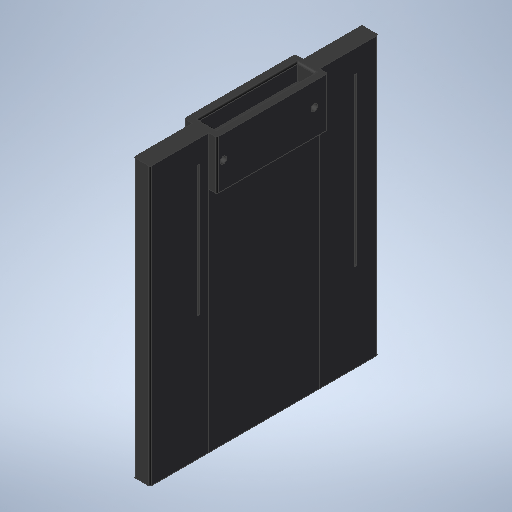
# Autodesk Inventor part: Chassis_Lower_Portion
Saved by Autodesk Inventor 2025 (Build 290162000, 162)
## iProperties
Created: 2024-06-26
Part Number: Chassis_Lower_Portion
Material: Generic
Document SubType Name: Modeling
Designer: sml6042
Density: 1 g/cm^3
Appearance: Default
Author: sml6042
Autodesk Inventor part; units mm, degrees
ref_plane "YZ Plane" through (0, 0, 0) normal (1, 0, 0) x (0, 1, 0)
ref_plane "XZ Plane" through (0, 0, 0) normal (0, 1, 0) x (-1, 0, 0)
ref_plane "XY Plane" through (0, 0, 0) normal (0, 0, 1) x (1, 0, 0)
sketch "Sketch1" plane through (0, 0, 0) normal (1, 0, 0) x (0, 1, 0)
  line L0 (0, 0) -> (0, -70)
  line L1 (0, -70) -> (-85, -70)
  line L2 (-85, -70) -> (-85, 0)
  line L3 (-85, 0) -> (0, 0)
  dimension "d0" = 70
  dimension "d1" = 85
  constraints: 8 end point, 3 perpendicular, 1 vertical
  measures "d0" distance of L0.start L0.end
  measures "d1" distance of L0.end L1.end
extrude "Extrusion1" add sketch "Sketch1" along normal blind 10
sketch "Sketch2" plane through (0, 0, 0) normal (0, 1, 0) x (1, 0, 0)
  line L0 (0, 0) -> (0, 70) projected
  line L1 (0, 0) -> (0, 20.125)
  line L2 (0, 20.125) -> (2.38, 20.125)
  line L3 (2.38, 20.125) -> (2.38, 50.375)
  line L4 (2.38, 50.375) -> (7.63, 50.375)
  line L5 (7.63, 50.375) -> (7.63, 20.125)
  line L6 (7.63, 20.125) -> (2.38, 20.125)
  dimension "d4" = 20.125
  dimension "d5" = 2.38
  dimension "d6" = 30.25
  dimension "d7" = 5.25
  constraints: 12 end point, 4 perpendicular, 2 point on line, 1 horizontal
  measures "d4" distance of L0.start L1.end
  measures "d5" distance of L1.end L2.end
  measures "d6" distance of L2.end L3.end
  measures "d7" distance of L3.end L4.end
extrude "Extrusion2" cut sketch "Sketch2" against normal blind 5.1
sketch "Sketch3" plane through (0, 0, 0) normal (-1, 0, 0) x (0, 0, 1)
  line L0 (0, 0) -> (0, -85) projected
  line L1 (0, 0) -> (-20, 0)
  line L2 (-70, 0) -> (0, 0) projected
  line L3 (-20, 0) -> (-20, -7)
  circle A0 centre (-20, -7) radius 1.025
  circle A1 centre (-47.9, -7) radius 1.025
  line L4 (-20, -7) -> (-14.9, -7)
  line L5 (-14.9, -7) -> (-14.6, -7)
  line L6 (-14.6, -7) -> (-14.6, -47)
  line L7 (-14.6, -47) -> (-15.2, -47)
  line L8 (-15.2, -47) -> (-15.2, -7)
  line L9 (-15.2, -7) -> (-14.6, -7)
  line L10 (-20, -7) -> (-21.025, -7)
  line L11 (-46.875, -7) -> (-47.9, -7)
  line L12 (-47.9, -7) -> (-63.1, -7)
  line L13 (-63.1, -7) -> (-63.1, -47)
  line L14 (-63.1, -58) -> (-63.4, -58)
  line L15 (-63.4, -58) -> (-63.4, -7)
  line L16 (-63.4, -7) -> (-62.8, -7)
  line L17 (-62.8, -7) -> (-62.8, -58)
  line L18 (-62.8, -58) -> (-63.1, -58)
  line L19 (-47.9, -7) -> (-20, -7)
  line L20 (-63.1, -47) -> (-63.1, -58)
  line L21 (-70, -85) -> (-70, 0) projected
  line L22 (-63.1, -58) -> (-62.8, -58)
  line L23 (-62.8, -58) -> (-62.8, -7)
  line L24 (-63.4, -7) -> (-62.8, -7)
  dimension "d12" = 2.05
  dimension "d14" = 2.05
  dimension "d10" = 20
  dimension "d11" = 7
  dimension "d13" = 27.9
  dimension "d17" = 5.1
  dimension "d18" = 0.3
  dimension "d19" = 40
  dimension "d20" = 0.6
  dimension "d21" = 40
  dimension "d22" = 15.2
  dimension "d23" = 51
  dimension "d24" = 0.3
  dimension "d25" = 0.6
  dimension "d26" = 51
  constraints: 44 end point, 6 horizontal, 6 perpendicular, 6 point on line, 2 coincident, 2 horizontal alignment, 2 parallel, 1 collinear, 4 other
  measures "d10" distance of L0.start L1.end
  measures "d11" distance of L1.end L3.end
  measures "d13" distance of L4.start L11.end
  measures "d17" distance of L4.start L4.end
  measures "d18" distance of L4.end L5.end
  measures "d19" distance of L5.end L6.end
  measures "d20" distance of L6.end L7.end
  measures "d21" distance of L7.end L8.end
  measures "d22" distance of L12.start L12.end
  measures "d23" distance of L12.end L14.start
  measures "d24" distance of L14.start L14.end
  measures "d25" distance of L15.end L16.end
  measures "d26" distance of L16.end L17.end
extrude "Extrusion3" cut sketch "Sketch3" against normal blind 10 contours A0 L4 L3 | A1 L12 L11 | L11 L12 A1 | L3 L10 A0 | L4 A0 L10
sketch "Sketch4" plane through (0, 0, 0) normal (-1, 0, 0) x (0, 0, 1)
  circle A0 centre (-19.9999, -6.9744) radius 1.25
  circle A1 centre (-47.8999, -6.9744) radius 1.25
  line L0 (-19.9999, -6.9744) -> (-14.8999, -6.9744)
  line L1 (-14.8999, -6.9744) -> (-14.5999, -6.9744)
  line L2 (-14.5999, -6.9744) -> (-14.5999, -46.9744)
  line L3 (-14.5999, -46.9744) -> (-15.1999, -46.9744)
  line L4 (-15.1999, -46.9744) -> (-15.1999, -6.9744)
  line L5 (-15.1999, -6.9744) -> (-14.5999, -6.9744)
  line L6 (-19.9999, -6.9744) -> (-21.2499, -6.9744)
  line L7 (-46.6499, -6.9744) -> (-47.8999, -6.9744)
  line L8 (-47.8999, -6.9744) -> (-63.0999, -6.9744)
  line L9 (-63.0999, -6.9744) -> (-63.0999, -46.9744)
  line L10 (-63.0999, -57.9744) -> (-63.3999, -57.9744)
  line L11 (-63.3999, -57.9744) -> (-63.3999, -6.9744)
  line L12 (-63.3999, -6.9744) -> (-62.7999, -6.9744)
  line L13 (-62.7999, -6.9744) -> (-62.7999, -57.9744)
  line L14 (-62.7999, -57.9744) -> (-63.0999, -57.9744)
  line L15 (-47.8999, -6.9744) -> (-19.9999, -6.9744)
  line L16 (-63.0999, -46.9744) -> (-63.0999, -57.9744)
  line L17 (-63.0999, -57.9744) -> (-62.7999, -57.9744)
  line L18 (-62.7999, -57.9744) -> (-62.7999, -6.9744)
  line L19 (-63.3999, -6.9744) -> (-62.7999, -6.9744)
  point P0 (0, 0)
  dimension "d27" = 2.5
  dimension "d29" = 2.5
  dimension "d28" = 27.9
  dimension "d30" = 5.1
  dimension "d31" = 0.3
  dimension "d32" = 40
  dimension "d33" = 0.6
  dimension "d34" = 40
  dimension "d35" = 15.2
  dimension "d36" = 51
  dimension "d37" = 0.3
  dimension "d38" = 0.6
  dimension "d39" = 51
  constraints: 40 end point, 6 horizontal, 5 perpendicular, 5 point on line, 2 coincident, 2 horizontal alignment, 1 collinear, 1 parallel, 4 other
  measures "d28" distance of L15.end L7.end
  measures "d30" distance of L15.end L0.end
  measures "d31" distance of L0.end L5.end
  measures "d32" distance of L5.end L3.start
  measures "d33" distance of L3.start L4.start
  measures "d34" distance of L4.start L5.start
  measures "d35" distance of L15.start L8.end
  measures "d36" distance of L8.end L14.end
  measures "d37" distance of L14.end L10.end
  measures "d38" distance of L19.start L19.end
  measures "d39" distance of L19.end L13.end
extrude "Extrusion4" cut sketch "Sketch4" against normal blind 10 contours L13 L14 L16 L9 L8 | L0 L1 L2 L3 L4 | L9 L16 L10 L11 L12
sketch "Sketch5" plane through (0, 0, 0) normal (0, 1, 0) x (1, 0, 0)
  line L0 (0, 0) -> (10, 0) projected
  line L1 (0, 0) -> (2.5, 0)
  line L2 (2.5, 0) -> (2.5, 18)
  line L3 (2.5, 18) -> (0, 18)
  line L4 (0, 70) -> (0, 0) projected
  line L5 (10, 0) -> (7.5, 0)
  line L6 (7.5, 0) -> (7.5, 18)
  line L7 (7.5, 18) -> (10, 18)
  line L8 (10, 70) -> (10, 0) projected
  line L9 (10, 0) -> (10, 18)
  line L10 (7.5, 0) -> (7.5, 18)
  line L11 (10, 18) -> (10, 0)
  line L12 (0, 18.975) -> (10, 18.975) projected
  line L13 (10, 70) -> (10, 52)
  line L14 (10, 52) -> (7.5003, 52)
  line L15 (7.5003, 52) -> (7.5003, 70)
  line L16 (7.5003, 70) -> (10, 70)
  line L17 (10, 70) -> (10, 52)
  line L18 (10, 70) -> (10, 52)
  line L19 (0, 70) -> (0, 52)
  line L20 (0, 52) -> (2.5, 52)
  line L21 (2.5, 52) -> (2.5, 70)
  line L22 (2.5, 70) -> (0, 70)
  dimension "d42" = 2.5
  dimension "d43" = 18
  dimension "d44" = 2.5
  dimension "d45" = 18
  dimension "d46" = 18
  dimension "d47" = 18
  constraints: 38 end point, 9 perpendicular, 9 point on line, 3 collinear, 2 horizontal
  measures "d42" distance of L0.start L1.end
  measures "d43" distance of L1.end L2.end
  measures "d44" distance of L5.start L5.end
  measures "d45" distance of L5.end L6.end
  measures "d46" distance of L8.start L13.end
  measures "d47" distance of L4.start L19.end
extrude "Extrusion5" cut sketch "Sketch5" against normal through all contours L4 L3 L2 L0 | L4 L22 L21 L20 | L14 L15 L16 L8 | L6 L7 L8 L0
sketch "Sketch6" plane through (0, -85, -52) normal (0, -1, 0) x (1, 0, 0)
  line L0 (2.5, 34) -> (2.5, 52) projected
  line L1 (2.5, 0) -> (2.5, 34)
  line L2 (2.5, 34) -> (0, 34)
  line L3 (0, 0) -> (0, 34) projected
  line L4 (0, 34) -> (0, 0)
  line L5 (0, 0) -> (2.5, 0)
  line L6 (7.5003, 0) -> (7.5003, 34)
  line L7 (10.0003, 34) -> (10.0003, 0)
  line L8 (10.0003, 0) -> (7.5003, 0)
  line L9 (7.5003, -18) -> (7.5003, 0) projected
  line L10 (7.5, 52) -> (7.5, 34) projected
  line L11 (7.5, 34) -> (7.5, 4)
  line L12 (7.5, 4) -> (7.5003, 0)
  line L13 (7.5, 34) -> (10, 34) projected
  line L14 (7.5, 34) -> (10, 34)
  point P0 (0, 52)
  dimension "d52" = 2.5
  dimension "d53" = 30
  constraints: 20 end point, 5 perpendicular, 4 point on line, 3 collinear, 1 parallel
  measures "d52" distance of L6.start L7.end
  measures "d53" distance of L10.end L11.end
extrude "Extrusion6" cut sketch "Sketch6" against normal blind 70 contours L5 L3 L2 L1
sketch "Sketch7" plane through (2.5, -85, -70) normal (0, -1, 0) x (1, 0, 0)
  line L0 (5, 52) -> (7.5, 52) projected
  line L1 (5.0003, 18) -> (5, 52)
  line L2 (5, 52) -> (7.5, 52)
  line L3 (7.5, 52) -> (7.5, 18)
  line L4 (7.5, 18) -> (5.0003, 18)
  point P0 (-2.5, 70)
  constraints: 8 end point, 2 perpendicular, 1 collinear
extrude "Extrusion7" cut sketch "Sketch7" against normal blind 70
fillet "Fillet1" radius 0.5 11 edges at (7.5003, -42.5, -70) (2.5, -42.5, 0) (7.5, -42.5, 0) (10, -7.5, -18) (10, -7.5, -52) (0, -7.5, -18) (0, -7.5, -52) (7.63, 0, -35.25) (2.38, 0, -35.25) (5.005, 0, -20.125) (5.005, 0, -50.375)
body "Solid1"
